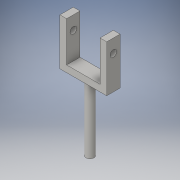
# Autodesk Inventor part: TopFork
Saved by Autodesk Inventor 2016 (Build 200138000, 138)
## iProperties
Created: 2017-04-12
Part Number: TopFork
Material: Generic
Document SubType Name: Modeling
Designer: Evan Phil George
Density: 1 g/cm^3
Appearance: Default
Author: Evan Phil George
Autodesk Inventor part; units mm, degrees
ref_plane "YZ Plane" through (0, 0, 0) normal (1, 0, 0) x (0, 1, 0)
ref_plane "XZ Plane" through (0, 0, 0) normal (0, 1, 0) x (-1, 0, 0)
ref_plane "XY Plane" through (0, 0, 0) normal (0, 0, 1) x (1, 0, 0)
sketch "Sketch1" plane through (0, 0, 0) normal (0, 0, 1) x (1, 0, 0)
  line L0 (0, 0) -> (12.5, 0)
  line L1 (12.5, 0) -> (12.5, 30)
  line L2 (12.5, 30) -> (17.5, 30)
  line L3 (17.5, 30) -> (17.5, -5)
  line L4 (17.5, -5) -> (-17.5, -5)
  line L5 (-17.5, -5) -> (-17.5, 30)
  line L6 (-17.5, 30) -> (-12.5, 30)
  line L7 (-12.5, 30) -> (-12.5, 0)
  line L8 (-12.5, 0) -> (12.5, 0)
  dimension "d0" = 12.5
  dimension "d1" = 30
  dimension "d2" = 5
  dimension "d3" = 35
  dimension "d4" = 35
  dimension "d5" = 35
  dimension "d6" = 5
  dimension "d8" = 30
  constraints: 18 end point, 4 perpendicular, 2 point on line, 1 horizontal, 1 vertical
  measures "d0" distance of L0.start L0.end
  measures "d1" distance of L0.end L1.end
  measures "d2" distance of L1.end L2.end
  measures "d3" distance of L2.end L3.end
  measures "d4" distance of L3.end L4.end
  measures "d5" distance of L4.end L5.end
  measures "d6" distance of L5.end L6.end
  measures "d8" distance of L6.end L7.end
extrude "Extrusion1" add sketch "Sketch1" along normal blind 10
sketch "Sketch2" plane through (-17.5, -5, 0) normal (0, -1, 0) x (1, 0, 0)
  line L0 (5, 10) -> (0, 10) projected
  line L1 (30, 0) -> (35, 0) projected
  line L2 (0, 10) -> (35, 0)
  circle A0 centre (17.5, 5) radius 3
  point P0 (17.5, 0)
  dimension "d11" = 6
  constraints: 2 end point, 1 centre point, 1 midpoint
  measures "d11" diameter of A0
extrude "Extrusion2" add sketch "Sketch2" along normal blind 50
sketch "Sketch3" plane through (-17.5, -5, 0) normal (-1, 0, 0) x (0, 0, 1)
  line L0 (0, 35) -> (10, 35) projected
  line L1 (5, 35) -> (5, 25)
  circle A0 centre (5, 25) radius 2.5
  point P0 (0, 5)
  dimension "d14" = 10
  dimension "d15" = 5
  constraints: 2 end point, 1 centre point, 1 coincident, 1 midpoint, 1 vertical
  measures "d14" distance of L1.start L1.end
  measures "d15" diameter of A0
extrude "Extrusion3" cut sketch "Sketch3" against normal blind 35
body "Solid1"
